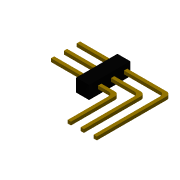
# Autodesk Inventor part: HeaderRight3
Saved by Autodesk Inventor 2015 (Build 190159000, 159)
## iProperties
Created: 2014-08-02
Part Number: HeaderRight3
Material: Generic
Document SubType Name: Modeling
Designer: david
Density: 1 g/cm^3
Appearance: Black
Author: david
Autodesk Inventor part; units mm, degrees
ref_plane "YZ Plane" through (0, 0, 0) normal (1, 0, 0) x (0, 1, 0)
ref_plane "XZ Plane" through (0, 0, 0) normal (0, 1, 0) x (-1, 0, 0)
sketch "Sketch1" plane through (0, 0, 0) normal (0, 1, 0) x (-1, 0, 0)
  line L0 (2.5467, 7.6401) -> (1.9117, 7.6401)
  line L1 (1.9117, 7.6401) -> (1.9117, -1.0276)
  line L2 (2.7055, -1.8214) -> (14.6752, -1.8214)
  line L3 (14.6752, -1.8214) -> (14.6752, -1.1864)
  line L4 (14.6752, -1.1864) -> (3.3405, -1.1864)
  line L5 (2.5467, 7.6401) -> (2.5467, -0.3926)
  line L6 (-0.6283, 7.6401) -> (-0.6283, -3.5676)
  line L7 (0.1655, -4.3614) -> (14.6752, -4.3614)
  line L8 (14.6752, -4.3614) -> (14.6752, -3.7264)
  line L9 (14.6752, -3.7264) -> (0.8005, -3.7264)
  line L10 (0.0067, -2.9326) -> (0.0067, 7.6401)
  line L11 (0.0067, 7.6401) -> (-0.6283, 7.6401)
  line L12 (-2.5333, 7.6401) -> (-3.1683, 7.6401)
  line L13 (-3.1683, 7.6401) -> (-3.1683, -6.1076)
  line L14 (-2.3745, -6.9014) -> (14.6752, -6.9014)
  line L15 (14.6752, -6.9014) -> (14.6752, -6.2664)
  line L16 (14.6752, -6.2664) -> (-1.7395, -6.2664)
  line L17 (-2.5333, -5.4726) -> (-2.5333, 7.6401)
  line L18 (14.6752, -1.5039) -> (20.4389, -1.5039) construction
  line L19 (14.6752, -4.0439) -> (20.4389, -4.0439) construction
  line L20 (14.6752, -6.5839) -> (20.223, -6.5839) construction
  line L21 (2.2292, 7.6401) -> (2.2292, 18.3973) construction
  line L22 (-0.3108, 7.6401) -> (-0.3108, 17.4615) construction
  line L23 (-2.8508, 7.6401) -> (-2.8508, 17.4615) construction
  line L24 (8.8332, 0.2741) -> (6.2932, 0.2741) construction
  line L25 (6.2932, 0.2741) -> (6.2932, -7.8285) construction
  line L26 (6.2932, -7.8285) -> (8.8332, -7.8285) construction
  line L27 (8.8332, -7.8285) -> (8.8332, 0.2741) construction
  arc A0 (2.5467, -0.3926) -> (3.3405, -1.1864) centre (3.3405, -0.3926) ccw
  arc A1 (1.9117, -1.0276) -> (2.7055, -1.8214) centre (2.7055, -1.0276) ccw
  arc A2 (0.0067, -2.9326) -> (0.8005, -3.7264) centre (0.8005, -2.9326) ccw
  arc A3 (-0.6283, -3.5676) -> (0.1655, -4.3614) centre (0.1655, -3.5676) ccw
  arc A4 (-2.5333, -5.4726) -> (-1.7395, -6.2664) centre (-1.7395, -5.4726) ccw
  arc A5 (-3.1683, -6.1076) -> (-2.3745, -6.9014) centre (-2.3745, -6.1076) ccw
  point P0 (0, 0)
  dimension "d2" = 0.635
  dimension "d3" = 2.54
  dimension "d4" = 2.54
  dimension "d5" = 2.54
  dimension "d6" = 2.54
  dimension "d7" = 8.1026
  dimension "d8" = 2.54
  dimension "d9" = 1.778
  dimension "d10" = 7.366
  dimension "d11" = 4.064
  dimension "d12" = 5.842
  dimension "d13" = 0.7937
  constraints: 56 end point, 13 perpendicular, 12 point on circle, 12 tangent, 7 horizontal, 6 centre point, 6 midpoint, 6 vertical, 5 equal length, 5 equal radius, 4 collinear, 2 parallel
  measures "d2" distance of L0.start L0.end
  measures "d3" distance between parallel lines of L22 L21
  measures "d4" distance between parallel lines of L23 L22
  measures "d5" distance between parallel lines of L19 L18
  measures "d6" distance between parallel lines of L20 L19
  measures "d7" distance of L26.end L24.start
  measures "d8" distance of L25.end L26.end
  measures "d9" distance between parallel lines of L24 L18
  measures "d10" distance between parallel lines of L24 L0
  measures "d11" distance between parallel lines of L25 L21
  measures "d12" distance between parallel lines of L27 L3
  measures "d13" radius of A0
extrude "Extrusion1" add sketch "Sketch1" along normal mid plane 0.635
ref_plane "Work Plane1" through (-5.4042, -0.3175, 7.6401) normal (-1, 0, 0) x (0, 0, 1)
sketch "Sketch2" plane through (-5.4042, -0.3175, 7.6401) normal (-1, 0, 0) x (0, 0, 1)
  line L0 (-8.8265, 0) -> (-8.8265, 0.635) projected
  line L1 (-9.4615, 0.635) -> (-8.8265, 0.635) projected
  line L2 (-9.4615, 0) -> (-9.4615, 0.635) projected
  line L3 (-8.8265, 0) -> (-9.4615, 0) projected
  line L4 (-11.3665, 0) -> (-11.3665, 0.635) projected
  line L5 (-12.0015, 0.635) -> (-11.3665, 0.635) projected
  line L6 (-12.0015, 0) -> (-12.0015, 0.635) projected
  line L7 (-11.3665, 0) -> (-12.0015, 0) projected
  line L8 (-13.9065, 0) -> (-13.9065, 0.635) projected
  line L9 (-14.5415, 0.635) -> (-13.9065, 0.635) projected
  line L10 (-14.5415, 0) -> (-14.5415, 0.635) projected
  line L11 (-13.9065, 0) -> (-14.5415, 0) projected
  line L12 (-7.0485, -0.9525) -> (-15.1511, -0.9525)
  line L13 (-15.1511, -0.9525) -> (-15.1511, 1.5875)
  line L14 (-15.1511, 1.5875) -> (-7.0485, 1.5875)
  line L15 (-7.0485, 1.5875) -> (-7.0485, -0.9525)
  line L16 (-9.144, 0) -> (-9.144, -1.4837) construction
  line L17 (-11.684, 0) -> (-11.684, -1.596) construction
  line L18 (-14.224, 0) -> (-14.224, -1.596) construction
  line L19 (-14.5415, 0.3175) -> (-17.2072, 0.3175) construction
  point P0 (-7.6401, 0.3175)
  point P1 (-15.1511, 0.3175)
  dimension "d17" = 8.1026
  dimension "d18" = 1.778
  dimension "d19" = 2.54
  constraints: 16 end point, 5 midpoint, 3 vertical, 2 horizontal, 2 parallel, 1 perpendicular, 1 point on line
  measures "d17" distance between parallel lines of L13 L15
  measures "d18" distance between parallel lines of L15 L0
  measures "d19" distance of L12.end L13.end
extrude "Extrusion2" add sketch "Sketch2" along normal blind 2.54
body "Solid1"
